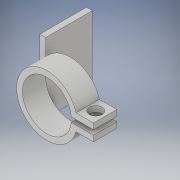
# Autodesk Inventor part: Ultrasonic Mount
Saved by Autodesk Inventor 2017 (Build 210142000, 142)
## iProperties
Created: 2018-01-09
Part Number: Ultrasonic Mount
Material: Generic
Document SubType Name: Modeling
Designer: prakh
Density: 1 g/cm^3
Appearance: Default
Author: prakh
Autodesk Inventor part; units mm, degrees
ref_plane "YZ Plane" through (0, 0, 0) normal (1, 0, 0) x (0, 1, 0)
ref_plane "XZ Plane" through (0, 0, 0) normal (0, 1, 0) x (-1, 0, 0)
ref_plane "XY Plane" through (0, 0, 0) normal (0, 0, 1) x (1, 0, 0)
sketch "Sketch1" plane through (0, 0, 0) normal (0, 0, 1) x (1, 0, 0)
  arc A0 (13.2744, 1.27) -> (13.2744, -1.27) centre (0, 0) ccw
  line L0 (25.4, -4.445) -> (15.9004, -4.445)
  line L1 (6.1638, -4.445) -> (6.1638, -1.27)
  line L2 (13.2744, -1.27) -> (25.4, -1.27)
  line L3 (25.4, -1.27) -> (25.4, -4.445)
  line L4 (25.4, 1.27) -> (13.2744, 1.27)
  line L5 (8.3094, 1.6345) -> (8.3094, 4.8095)
  line L6 (25.4, 4.445) -> (25.4, 1.27)
  line L7 (15.9004, 4.445) -> (25.4, 4.445)
  arc A1 (15.9004, 4.445) -> (15.9004, -4.445) centre (0, 0) ccw
  dimension "d0" = 26.67
  dimension "d2" = 3.175
  dimension "d3" = 4.445
  dimension "d4" = 25.4
  dimension "d5" = 3.175
  constraints: 16 end point, 4 parallel, 4 point on circle, 2 centre point, 2 coincident, 2 equal length, 2 horizontal, 2 perpendicular, 1 collinear
  measures "d0" diameter of A0
  measures "d2" distance of L2.end L0.start
  measures "d3" distance from line of point (0, 0) L0
  measures "d4" distance from line of point (0, 0) L3
  measures "d5" radial gap between concentric circles of A0 A1
extrude "Extrusion1" add sketch "Sketch1" along normal blind 12.7
sketch "Sketch2" plane through (15.9004, 4.445, 0) normal (0, 1, 0) x (1, 0, 0)
  circle A0 centre (4.4196, -6.35) radius 2.4638
  line L0 (9.4996, -12.7) -> (0, -12.7) projected
  line L1 (9.4996, 0) -> (9.4996, -12.7) projected
  point P0 (-15.9004, 0)
  dimension "d8" = 6.35
  dimension "d9" = 5.08
  dimension "d10" = 4.9276
  constraints: 1 centre point
  measures "d8" distance from line of A0.centre L0
  measures "d9" distance from line of A0.centre L1
  measures "d10" diameter of A0
extrude "Extrusion2" cut sketch "Sketch2" against normal blind 25.4
sketch "Sketch3" plane through (15.9004, 4.445, 0) normal (0, 1, 0) x (1, 0, 0)
  circle A0 centre (4.4196, -6.35) radius 2.4638 projected
  circle A1 centre (4.4196, -6.35) radius 3.4798
  point P0 (-15.9004, 0)
  dimension "d13" = 1.016
  constraints: 1 centre point, 1 coincident
  measures "d13" radial gap between concentric circles of A0 A1
extrude "Extrusion3" cut sketch "Sketch3" against normal up to surface (3.175 mm away)
sketch "Sketch4" plane through (0, 0, 0) normal (0, 0, -1) x (-1, 0, 0)
  line L0 (16.51, -19.05) -> (13.335, -19.05)
  line L1 (13.335, -19.05) -> (13.335, 19.05)
  line L2 (13.335, 19.05) -> (16.51, 19.05)
  line L3 (16.51, 19.05) -> (16.51, -19.05)
  arc A0 (-13.2744, -1.27) -> (-13.2744, 1.27) centre (0, 0) ccw projected
  arc A1 (-15.9004, -4.445) -> (-15.9004, 4.445) centre (0, 0) ccw projected
  dimension "d16" = 19.05
  dimension "d17" = 19.05
  constraints: 8 end point, 2 parallel, 2 tangent, 1 horizontal, 1 perpendicular
  measures "d16" distance from line of point (0, 0) L2
  measures "d17" distance from line of point (0, 0) L0
extrude "Extrusion4" add sketch "Sketch4" along normal blind 25.4
equation "\"d17\" = d16"
body "Solid1"
